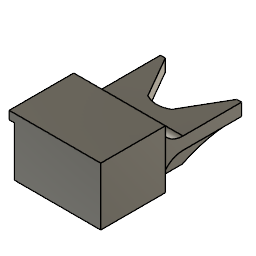
workout-dumbbell-holder (Autodesk Fusion 360 design; units mm, degrees)
Autodesk Fusion 360 part; units mm, degrees
ref_plane "WorkPlane1" through (0, 0, -38) normal (0, 0, 1) x (1, 0, 0)
sketch "Sketch1" plane through (0, 0, -38) normal (0, 0, 1) x (1, 0, 0)
  line L0 (-34.25, -21.25) -> (34.25, -21.25)
  line L1 (34.25, -21.25) -> (34.25, 21.25)
  line L2 (34.25, 21.25) -> (-34.25, 21.25)
  line L3 (-34.25, 21.25) -> (-34.25, -21.25)
extrude "Extrude1" add sketch "Sketch1" along normal blind 30
fillet "Fillet1" radius 2.5 4 edges at (-34.25, 21.25, -23) (34.25, 21.25, -23) (34.25, -21.25, -23) (-34.25, -21.25, -23)
ref_plane "WorkPlane2" through (0, 0, -8) normal (0, 0, 1) x (1, 0, 0)
sketch "Sketch2" plane through (0, 0, -8) normal (0, 0, 1) x (1, 0, 0)
  line L0 (-44.25, -31.25) -> (44.25, -31.25)
  line L1 (44.25, -31.25) -> (44.25, 31.25)
  line L2 (44.25, 31.25) -> (-44.25, 31.25)
  line L3 (-44.25, 31.25) -> (-44.25, -31.25)
extrude "Extrude2" add sketch "Sketch2" along normal blind 8
ref_plane "WorkPlane3" through (0, 0, -38) normal (0, 0, 1) x (1, 0, 0)
sketch "Sketch3" plane through (0, 0, -38) normal (0, 0, 1) x (1, 0, 0)
  line L0 (-44.25, -31.25) -> (44.25, -31.25)
  line L1 (44.25, -31.25) -> (44.25, 31.25)
  line L2 (44.25, 31.25) -> (-44.25, 31.25)
  line L3 (-44.25, 31.25) -> (-44.25, -31.25)
  line L4 (-39.25, -26.5) -> (39.25, -26.5)
  line L5 (39.25, -26.5) -> (39.25, 26.5)
  line L6 (39.25, 26.5) -> (-39.25, 26.5)
  line L7 (-39.25, 26.5) -> (-39.25, -26.5)
extrude "Extrude3" add sketch "Sketch3" along normal blind 30
ref_plane "WorkPlane4" through (0, 0, -34) normal (0, 0, 1) x (1, 0, 0)
sketch "Sketch4" plane through (0, 0, -34) normal (0, 0, 1) x (1, 0, 0)
  line L0 (-44.25, 26.5) -> (44.25, 26.5)
  line L1 (44.25, 26.5) -> (44.25, 110)
  line L2 (44.25, 110) -> (-44.25, 110)
  line L3 (-44.25, 110) -> (-44.25, 26.5)
extrude "Extrude4" add sketch "Sketch4" along normal blind 12
sketch "Sketch5" plane through (0, 0, -34) normal (0, 0, 1) x (1, 0, 0)
  line L0 (-34.547, 110) -> (-11.5, 70.0814)
  arc A0 (-11.5, 70.0814) -> (11.5, 70.0814) centre (0, 90) ccw
  line L1 (11.5, 70.0814) -> (34.547, 110)
  line L2 (34.547, 110) -> (34.547, 115)
  line L3 (34.547, 115) -> (-34.547, 115)
  line L4 (-34.547, 115) -> (-34.547, 110)
extrude "Extrude5" cut sketch "Sketch5" along normal blind 12
fillet "Fillet2" radius 5 64 edges at (33.5178, -20.5178, -8) (0, -21.25, -8) (-33.5178, -20.5178, -8) (-34.25, 0, -8) (-33.5178, 20.5178, -8) (0, 21.25, -8) (33.5178, 20.5178, -8) (34.25, 0, -8) (34.25, 0, -8) (33.5178, 20.5178, -8) (0, 21.25, -8) (-33.5178, 20.5178, -8) (-34.25, 0, -8) (-33.5178, -20.5178, -8) (0, -21.25, -8) (33.5178, -20.5178, -8) (33.5178, 20.5178, -8) (34.25, 0, -8) (33.5178, -20.5178, -8) (0, -21.25, -8) (-33.5178, -20.5178, -8) (-34.25, 0, -8) (-33.5178, 20.5178, -8) (0, 21.25, -8) (0, 21.25, -8) (-33.5178, 20.5178, -8) (-34.25, 0, -8) (-33.5178, -20.5178, -8) (0, -21.25, -8) (33.5178, -20.5178, -8) (34.25, 0, -8) (33.5178, 20.5178, -8) (-33.5178, 20.5178, -8) (0, 21.25, -8) (33.5178, 20.5178, -8) (34.25, 0, -8) (33.5178, -20.5178, -8) (0, -21.25, -8) (-33.5178, -20.5178, -8) (-34.25, 0, -8) (-34.25, 0, -8) (-33.5178, -20.5178, -8) (0, -21.25, -8) (33.5178, -20.5178, -8) (34.25, 0, -8) (33.5178, 20.5178, -8) (0, 21.25, -8) (-33.5178, 20.5178, -8) (-33.5178, -20.5178, -8) (-34.25, 0, -8) (-33.5178, 20.5178, -8) (0, 21.25, -8) (33.5178, 20.5178, -8) (34.25, 0, -8) (33.5178, -20.5178, -8) (0, -21.25, -8) (0, -21.25, -8) (33.5178, -20.5178, -8) (34.25, 0, -8) (33.5178, 20.5178, -8) (0, 21.25, -8) (-33.5178, 20.5178, -8) (-34.25, 0, -8) (-33.5178, -20.5178, -8)
ref_plane "WorkPlane5" through (0, 0, -38) normal (0, 0, 1) x (1, 0, 0)
sketch "Sketch6" plane through (0, 0, -38) normal (0, 0, 1) x (1, 0, 0)
ref_plane "WorkPlane6" through (-39.25, 0, 0) normal (1, 0, 0) x (0, 1, 0)
sketch "Sketch8" plane through (-39.25, 0, 0) normal (1, 0, 0) x (0, 0, -1)
ref_plane "WorkPlane7" through (-39.25, 0, 0) normal (1, 0, 0) x (0, 1, 0)
sketch "Sketch9" plane through (-39.25, 0, 0) normal (1, 0, 0) x (0, 0, -1)
  line L0 (0, 31.25) -> (22, 31.25)
  line L1 (22, 31.25) -> (22, 53.25)
  arc A0 (0, 31.25) -> (22, 53.25) centre (0.0125, 53.2375) ccw
extrude "Extrude6" add sketch "Sketch9" along normal blind 83.5
ref_plane "WorkPlane8" through (0, 0, -38) normal (0, 0, 1) x (1, 0, 0)
sketch "Sketch10" plane through (0, 0, -38) normal (0, 0, 1) x (1, 0, 0)
  line L0 (-44.25, -31.25) -> (-39.25, -31.25)
  line L1 (-39.25, -31.25) -> (-39.25, 31.25)
  line L2 (-39.25, 31.25) -> (-44.25, 31.25)
  line L3 (-44.25, 31.25) -> (-44.25, -31.25)
extrude "Extrude7" cut sketch "Sketch10" along normal blind 30
ref_plane "WorkPlane9" through (0, 0, -56) normal (0, 0, 1) x (1, 0, 0)
sketch "Sketch11" plane through (0, 0, -56) normal (0, 0, 1) x (1, 0, 0)
  line L0 (-44.25, -31.25) -> (44.25, -31.25)
  line L1 (44.25, -31.25) -> (44.25, 31.25)
  line L2 (44.25, 31.25) -> (-44.25, 31.25)
  line L3 (-44.25, 31.25) -> (-44.25, -31.25)
  line L4 (-39.25, -26.5) -> (39.25, -26.5)
  line L5 (39.25, -26.5) -> (39.25, 26.5)
  line L6 (39.25, 26.5) -> (-39.25, 26.5)
  line L7 (-39.25, 26.5) -> (-39.25, -26.5)
extrude "Extrude8" add sketch "Sketch11" along normal blind 18
ref_plane "WorkPlane10" through (0, 0, -56) normal (0, 0, 1) x (1, 0, 0)
sketch "Sketch12" plane through (0, 0, -56) normal (0, 0, 1) x (1, 0, 0)
  line L0 (-44.25, -31.25) -> (-39.25, -31.25)
  line L1 (-39.25, -31.25) -> (-39.25, 31.25)
  line L2 (-39.25, 31.25) -> (-44.25, 31.25)
  line L3 (-44.25, 31.25) -> (-44.25, -31.25)
extrude "Extrude9" cut sketch "Sketch12" along normal blind 18
ref_plane "WorkPlane11" through (0, 0, -34) normal (0, 0, 1) x (1, 0, 0)
sketch "Sketch13" plane through (0, 0, -34) normal (0, 0, 1) x (1, 0, 0)
  line L0 (-44.25, 31.25) -> (-39.25, 31.25)
  line L1 (-39.25, 31.25) -> (-39.25, 110)
  line L2 (-39.25, 110) -> (-44.25, 110)
  line L3 (-44.25, 110) -> (-44.25, 31.25)
extrude "Extrude10" cut sketch "Sketch13" along normal blind 12
ref_plane "WorkPlane12" through (-39.25, 0, 0) normal (1, 0, 0) x (0, 1, 0)
sketch "Sketch14" plane through (-39.25, 0, 0) normal (1, 0, 0) x (0, 0, -1)
  line L0 (56, 31.25) -> (34, 31.25)
  line L1 (34, 31.25) -> (34, 53.25)
  arc A0 (34, 53.25) -> (56, 31.25) centre (55.9875, 53.2375) ccw
extrude "Extrude11" add sketch "Sketch14" along normal blind 83.5
ref_plane "WorkPlane13" through (0, 0, -46) normal (0, 0, 1) x (1, 0, 0)
sketch "Sketch15" plane through (0, 0, -46) normal (0, 0, 1) x (1, 0, 0)
  line L0 (-38.5, 31.25) -> (-35.5, 31.25)
  line L1 (-35.5, 31.25) -> (-35.5, 105)
  line L2 (-35.5, 105) -> (-38.5, 105)
  line L3 (-38.5, 105) -> (-38.5, 31.25)
  line L4 (35.5, 31.25) -> (38.5, 31.25)
  line L5 (38.5, 31.25) -> (38.5, 105)
  line L6 (38.5, 105) -> (35.5, 105)
  line L7 (35.5, 105) -> (35.5, 31.25)
extrude "Extrude12" add sketch "Sketch15" along normal blind 12
ref_plane "WorkPlane14" through (35.5, 0, 0) normal (1, 0, 0) x (0, 1, 0)
sketch "Sketch16" plane through (35.5, 0, 0) normal (1, 0, 0) x (0, 0, -1)
  arc A0 (34, 105) -> (46, 53.25) centre (151.5034, 104.9809) ccw
  line L0 (34, 105) -> (46, 105)
  line L1 (46, 105) -> (46, 53.25)
extrude "Extrude13" cut sketch "Sketch16" along normal blind 3
ref_plane "WorkPlane15" through (-38.5, 0, 0) normal (1, 0, 0) x (0, 1, 0)
sketch "Sketch17" plane through (-38.5, 0, 0) normal (1, 0, 0) x (0, 0, -1)
  arc A0 (34, 105) -> (46, 53.25) centre (151.5034, 104.9809) ccw
  line L0 (34, 105) -> (46, 105)
  line L1 (46, 105) -> (46, 53.25)
extrude "Extrude14" cut sketch "Sketch17" along normal blind 3
ref_plane "WorkPlane16" through (0, 0, -56) normal (0, 0, 1) x (1, 0, 0)
sketch "Sketch18" plane through (0, 0, -56) normal (0, 0, 1) x (1, 0, 0)
  line L0 (39.25, 31.25) -> (44.25, 31.25)
  line L1 (44.25, 31.25) -> (44.25, 110)
  line L2 (44.25, 110) -> (39.25, 110)
  line L3 (39.25, 110) -> (39.25, 31.25)
extrude "Extrude15" cut sketch "Sketch18" along normal blind 56
named bodies: "holder"
